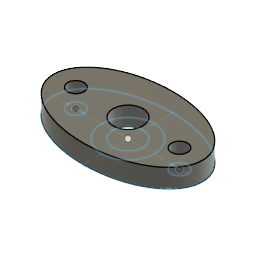
Assembled Box (Autodesk Fusion 360 archive; units mm, degrees)
design "Elllipse"
part number: 2026-06-03-15-20-48-513
Autodesk Fusion 360 part; units mm, degrees
sketch "Sketch1" plane through (0, 0, 0) normal (0, 1, 0) x (1, 0, 0)
sketch "Sketch2" plane through (0, 15, 0) normal (0, 1, 0) x (-1, 0, 0)
sketch "Sketch3" plane through (0, 15, 0) normal (0, 1, 0) x (-1, 0, 0)
  ellipse E0 centre (250.1558, -249.9936) end of major axis (250.1558, -285.9936) minor radius 60
  line L0 (250.1558, -213.9936) -> (250.1558, -285.9936) construction
  line L1 (190.1558, -249.9936) -> (310.1558, -249.9936) construction
  line L2 (214.6588, -249.4953) -> (208.1588, -249.4953)
  circle A0 centre (208.1588, -249.4953) radius 6.5
  line L3 (285.6558, -249.9936) -> (292.1558, -249.9936)
  circle A1 centre (292.1558, -249.9936) radius 6.5
  circle A2 centre (250.1558, -249.9936) radius 12
  circle A3 centre (250.1558, -249.9936) radius 21
  dimension "d14" = 72
  dimension "d15" = 120
  dimension "d16" = 42
  dimension "d17" = 13
  dimension "d18" = 42
  dimension "d19" = 13
  dimension "d24" = 24
  dimension "d25" = 42
  constraint coincident E0 L0.start
  constraint coincident E0 L0.end
  constraint coincident E0 L1.start
  constraint coincident E0 L1.end
  constraint vertical L0
  constraint perpendicular L0 L2
  constraint coincident L2.end A0.centre
  constraint perpendicular L0 L3
  constraint coincident L3.end A1.centre
  constraint coincident A1 L3.start
  constraint coincident A0 L2.start
  constraint concentric E0 A2
  constraint concentric E0 A3
  measures "d14" distance of E0
  measures "d16" distance of E0.centre L2.end
  measures "d17" diameter of A0
  measures "d18" distance of E0.centre L3.end
  measures "d19" diameter of A1
  measures "d24" diameter of A2
  measures "d25" diameter of A3
extrude "Extrude3" add sketch "Sketch3" along normal blind 15 contours E0 | A3
sketch "Sketch4" plane through (0, 0, 0) normal (0, 1, 0) x (1, 0, 0)
sketch "Sketch5" plane through (0, 0, 0) normal (0, 1, 0) x (1, 0, 0)

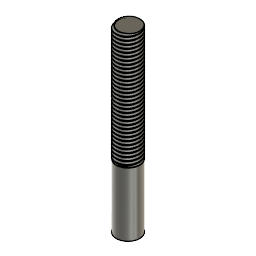
design "rod maker"
part number: 2026-06-04-10-37-24-051
Autodesk Fusion 360 part; units mm, degrees
sketch "Sketch1" plane through (0, 0, 0) normal (1, 0, 0) x (0, 1, 0)
sketch "Sketch2" plane through (0, 0, 0) normal (0, 0, 1) x (1, 0, 0)
sketch "Sketch3" plane through (0, 0, 0) normal (0, 0, 1) x (1, 0, 0)
  circle A0 centre (0, 0) radius 6
  dimension "d1" = 12
  constraint coincident A0.centre origin
  measures "d1" diameter of A0
extrude "Extrude1" add sketch "Sketch3" along normal blind 70
sketch "Sketch4" plane through (0, 0, 0) normal (1, 0, 0) x (0, 1, 0)
thread "Thread1" "ISO Metric profile 12.0 M12x1.75 M12x1.75 6g" major diameter 11.8335 minor diameter 9.8365 pitch 1.75 angle 60 modelled right hand crest width 0.2518 on face at (5.9702, -0.5974, 46.6667) from (0, 0, 12) to (0, 0, 70) crest through (5.9168, 0, -0.4375)
extrude "Extrude2" add 1 faces at (1.3581, 0.7601, 0) along direction (0, 0, -1) blind 20
named bodies: "rod maker"

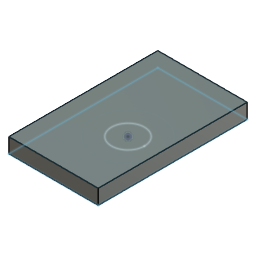
design "Bottom Plane"
part number: 2026-06-03-15-20-48-513
Autodesk Fusion 360 part; units mm, degrees
sketch "Sketch1" plane through (0, 0, 0) normal (0, 1, 0) x (1, 0, 0)
  line L0 (-45, 75) -> (-45, -75)
  line L1 (-45, -75) -> (45, -75)
  line L2 (45, -75) -> (45, 75)
  line L3 (45, 75) -> (-45, 75)
  circle A0 centre (0, 0) radius 16.5
  dimension "d9" = 33
  constraint perpendicular L0 L1
  constraint perpendicular L1 L2
  constraint coincident A0.centre origin
  measures "d9" diameter of A0
extrude "Extrude1" add sketch "Sketch1" along normal blind 15 contours L0 L1 L2 L3 | A0
move_face "MoveFace1" by (-220, 0, 0) 1 faces at (-15, 15, -25)
sketch "Sketch2" plane through (0, 15, 0) normal (0, 1, 0) x (-1, 0, 0)
  line L0 (-45, -75) -> (45, -75)
  line L1 (45, -75) -> (45, 75)
  line L2 (45, 75) -> (-45, 75)
  line L3 (-45, 75) -> (-45, -75)
sketch "Sketch3" plane through (0, 15, 0) normal (0, 1, 0) x (-1, 0, 0)
  line L0 (-45, -75) -> (45, -75)
  line L1 (45, -75) -> (45, 75)
  line L2 (45, 75) -> (-45, 75)
  line L3 (-45, 75) -> (-45, -75)
sketch "Sketch6" plane through (0, 30, 0) normal (0, 1, 0) x (-1, 0, 0)
sketch "Sketch10" plane through (0, 15, 0) normal (0, 1, 0) x (-1, 0, 0)
combine "Combine1" [no effect]
sketch "Sketch7" plane through (0, 15, 0) normal (0, 1, 0) x (-1, 0, 0)
sketch "Sketch8" plane through (0, 15, 0) normal (0, 1, 0) x (-1, 0, 0)
sketch "Sketch9" plane through (0, 15, 0) normal (0, 1, 0) x (-1, 0, 0)
extrude "Extrude3" [suppressed]
sketch "Sketch4" plane through (0, 0, 0) normal (0, 1, 0) x (1, 0, 0)
sketch "Sketch5" plane through (0, 0, 0) normal (0, 1, 0) x (1, 0, 0)
named bodies: "Body 1"

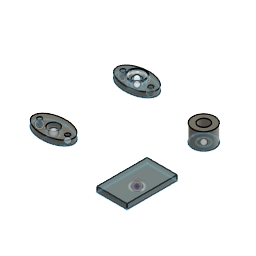
design "Stuffing Box"
part number: 2026-06-03-15-20-48-513
Autodesk Fusion 360 part; units mm, degrees
sketch "Sketch1" plane through (0, 0, 0) normal (0, 1, 0) x (1, 0, 0)
  line L0 (-45, 75) -> (-45, -75)
  line L1 (-45, -75) -> (45, -75)
  line L2 (45, -75) -> (45, 75)
  line L3 (45, 75) -> (-45, 75)
  circle A0 centre (0, 0) radius 16.5
  dimension "d9" = 33
  constraint perpendicular L0 L1
  constraint perpendicular L1 L2
  constraint coincident A0.centre origin
  measures "d9" diameter of A0
extrude "Extrude1" add sketch "Sketch1" along normal blind 15 contours L0 L1 L2 L3 | A0 makes body 1
move_face "MoveFace1" by (-220, 0, 0) 1 faces at (-15, 15, -25) on bodies 1
sketch "Sketch2" plane through (0, 15, 0) normal (0, 1, 0) x (-1, 0, 0)
  line L0 (-45, -75) -> (45, -75)
  line L1 (45, -75) -> (45, 75)
  line L2 (45, 75) -> (-45, 75)
  line L3 (-45, 75) -> (-45, -75)
  circle A0 centre (0, -200) radius 33
  circle A1 centre (0, -200) radius 16.5
  dimension "d10" = 66
  dimension "d11" = 33
  constraint concentric A0 A1
  measures "d10" diameter of A0
  measures "d11" diameter of A1
extrude "Extrude2" add sketch "Sketch2" along normal blind 50 separate body contours A0 makes body 2
sketch "Sketch3" plane through (0, 15, 0) normal (0, 1, 0) x (-1, 0, 0)
  line L0 (-45, -75) -> (45, -75)
  line L1 (45, -75) -> (45, 75)
  line L2 (45, 75) -> (-45, 75)
  line L3 (-45, 75) -> (-45, -75)
  ellipse E0 centre (250.1558, -249.9936) end of major axis (250.1558, -285.9936) minor radius 60
  line L4 (250.1558, -213.9936) -> (250.1558, -285.9936) construction
  line L5 (190.1558, -249.9936) -> (310.1558, -249.9936) construction
  line L6 (214.6588, -249.4953) -> (208.1588, -249.4953)
  circle A0 centre (208.1588, -249.4953) radius 6.5
  line L7 (285.6558, -249.9936) -> (292.1558, -249.9936)
  circle A1 centre (292.1558, -249.9936) radius 6.5
  ellipse E1 centre (250, 0) end of major axis (250, -36) minor radius 60
  line L8 (250, 36) -> (250, -36) construction
  line L9 (190, 0) -> (310, 0) construction
  circle A2 centre (250, 0) radius 16.5
  circle A3 centre (250.1558, -249.9936) radius 12
  circle A4 centre (250.1558, -249.9936) radius 21
  circle A5 centre (208, 0) radius 6.5
  line L10 (250, 0) -> (292, 0) construction
  circle A6 centre (292, 0) radius 6.5
  dimension "d14" = 72
  dimension "d15" = 120
  dimension "d16" = 42
  dimension "d17" = 13
  dimension "d18" = 42
  dimension "d19" = 13
  dimension "d20" = 72
  dimension "d21" = 120
  dimension "d22" = 42
  dimension "d23" = 33
  dimension "d24" = 24
  dimension "d25" = 42
  dimension "d41" = 13
  dimension "d48" = 42
  dimension "d49" = 13
  constraint coincident E0 L4.start
  constraint coincident E0 L4.end
  constraint coincident E0 L5.start
  constraint coincident E0 L5.end
  constraint vertical L4
  constraint perpendicular L4 L6
  constraint coincident L6.end A0.centre
  constraint perpendicular L4 L7
  constraint coincident L7.end A1.centre
  constraint coincident A1 L7.start
  constraint coincident A0 L6.start
  constraint coincident E1 L8.start
  constraint coincident E1 L8.end
  constraint coincident E1 L9.start
  constraint coincident E1 L9.end
  constraint vertical L8
  constraint concentric E1 A2
  constraint concentric E0 A3
  constraint concentric E0 A4
  constraint coincident E1.centre A2.centre
  constraint perpendicular L8 L10
  constraint coincident L10.end A6.centre
  measures "d14" distance of E0
  measures "d16" distance of E0.centre L6.end
  measures "d17" diameter of A0
  measures "d18" distance of E0.centre L7.end
  measures "d19" diameter of A1
  measures "d20" distance of E1
  measures "d22" distance of E1.centre A5.centre
  measures "d23" diameter of A2
  measures "d24" diameter of A3
  measures "d25" diameter of A4
  measures "d41" diameter of A5
  measures "d48" distance of E1.centre L10.end
  measures "d49" diameter of A6
extrude "Extrude4" add sketch "Sketch3" along normal blind 15 separate body contours E0 makes body 3
extrude "Extrude5" add sketch "Sketch3" along normal blind 9 separate body contours A4 makes body 4
extrude "Extrude6" add 1 faces at (-268.033, 24, -251.633) along direction (0, 1, 0) blind 6 on bodies 4 bodies 3 4
sketch "Sketch6" plane through (0, 30, 0) normal (0, 1, 0) x (-1, 0, 0)
  circle A0 centre (250.1558, -249.9936) radius 12
  circle A1 centre (208.1588, -249.4953) radius 6.5
  circle A2 centre (292.1558, -249.9936) radius 6.5
  ellipse E0 centre (250.1558, -249.9936) end of major axis (310.1558, -249.9936) minor radius 36
  circle A3 centre (250.1558, -249.9936) radius 25
  circle A4 centre (250.1558, -249.9936) radius 23
  dimension "d35" = 50
  dimension "d36" = 46
  constraint concentric A0 A3
  constraint concentric A3 A4
  measures "d35" diameter of A3
  measures "d36" diameter of A4
extrude "Extrude7" add sketch "Sketch6" along normal blind 9 contours A3 bodies 3
fillet "Fillet1" radius 13.5 1 edges at (-228.7123, 30, -258.3107) on bodies 3
sketch "Sketch10" plane through (0, 15, 0) normal (0, 1, 0) x (-1, 0, 0)
extrude "Extrude9" add sketch "Sketch3" along normal blind 15 separate body contours E0 makes body 5
extrude "Extrude10" add sketch "Sketch3" along normal blind 15 separate body contours E1 makes body 6
combine "Combine1" operation add target body 3 tool bodies 5
sketch "Sketch7" plane through (0, 15, 0) normal (0, 1, 0) x (-1, 0, 0)
  line L0 (250, 0) -> (292, 0) construction
  circle A0 centre (292, 0) radius 6.5
  dimension "d42" = 42
  dimension "d43" = 13
  constraint horizontal L0
  constraint coincident L0.end A0.centre
  measures "d42" distance of L0.start L0.end
  measures "d43" diameter of A0
sketch "Sketch8" plane through (0, 15, 0) normal (0, 1, 0) x (-1, 0, 0)
extrude "Extrude8" add sketch "Sketch3" along normal blind 15 separate body contours E1 | A6 makes body 7
sketch "Sketch9" plane through (0, 15, 0) normal (0, 1, 0) x (-1, 0, 0)
extrude "Extrude3" [suppressed]
sketch "Sketch4" plane through (0, 0, 0) normal (0, 1, 0) x (1, 0, 0)
sketch "Sketch5" plane through (0, 0, 0) normal (0, 1, 0) x (1, 0, 0)
named bodies: "Body 1", "Body 2", "Body 3", "Body 4"

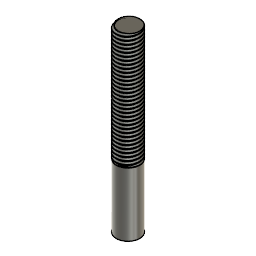
design "rod maker"
part number: 2026-06-04-10-37-24-051
Autodesk Fusion 360 part; units mm, degrees
sketch "Sketch1" plane through (0, 0, 0) normal (1, 0, 0) x (0, 1, 0)
sketch "Sketch2" plane through (0, 0, 0) normal (0, 0, 1) x (1, 0, 0)
sketch "Sketch3" plane through (0, 0, 0) normal (0, 0, 1) x (1, 0, 0)
  circle A0 centre (0, 0) radius 6
  dimension "d1" = 12
  constraint coincident A0.centre origin
  measures "d1" diameter of A0
extrude "Extrude1" add sketch "Sketch3" along normal blind 70
sketch "Sketch4" plane through (0, 0, 0) normal (1, 0, 0) x (0, 1, 0)
thread "Thread1" "ISO Metric profile 12.0 M12x1.75 M12x1.75 6g" major diameter 11.8335 minor diameter 9.8365 pitch 1.75 angle 60 modelled right hand crest width 0.2518 on face at (5.9702, -0.5974, 46.6667) from (0, 0, 12) to (0, 0, 70) crest through (5.9168, 0, -0.4375)
extrude "Extrude2" add 1 faces at (1.3581, 0.7601, 0) along direction (0, 0, -1) blind 20

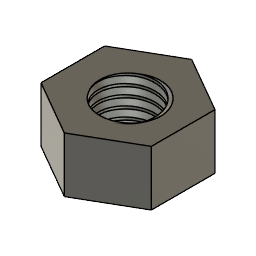
design "nut"
part number: 2026-06-04-11-31-36-315
Autodesk Fusion 360 part; units mm, degrees
sketch "Sketch1" plane through (0, 0, 0) normal (0, 0, 1) x (1, 0, 0)
  circle A0 centre (0, 0) radius 6
  line L0 (10, 5.7735) -> (0, 11.547)
  line L1 (0, 11.547) -> (-10, 5.7735)
  line L2 (-10, 5.7735) -> (-10, -5.7735)
  line L3 (-10, -5.7735) -> (0, -11.547)
  line L4 (0, -11.547) -> (10, -5.7735)
  line L5 (10, -5.7735) -> (10, 5.7735)
  dimension "d3" = 12
  constraint coincident A0.centre origin
  measures "d3" diameter of A0
extrude "Extrude1" add sketch "Sketch1" along normal blind 10
thread "Thread1" "ISO Metric profile 12.0 M12x1.75 M12x1.75 6H" major diameter 12.2265 minor diameter 10.2735 pitch 1.75 angle 60 modelled right hand crest width 0.4769 on face at (5.9925, -0.2991, 6.6667) crest through (5.1368, 0, 0.4375)

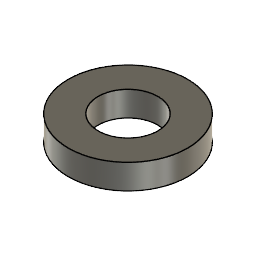
design "Screw"
part number: 2026-06-04-11-09-47-763
Autodesk Fusion 360 part; units mm, degrees
sketch "Sketch1" plane through (0, 0, 0) normal (1, 0, 0) x (0, 1, 0)
  line L0 (0, 0) -> (0, 5)
  line L1 (6, 0) -> (12, 0)
  line L2 (12, 0) -> (12, 5)
  line L3 (12, 5) -> (6, 5)
  line L4 (6, 5) -> (6, 0)
  dimension "d7" = 5
  dimension "d8" = 6
  constraint coincident L0.start origin
  constraint vertical L0
  constraint perpendicular L1 L2
  constraint perpendicular L2 L3
  measures "d7" distance of L0.start L0.end
  measures "d8" distance of L1.start L1.end
revolve "Revolve1" add sketch "Sketch1" angle 360 about axis through (0, 0, 0) along (0, 0, 1)
named bodies: "rod bottom cap"

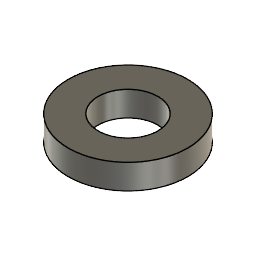
design "Screw"
part number: 2026-06-04-11-09-47-763
Autodesk Fusion 360 part; units mm, degrees
sketch "Sketch1" plane through (0, 0, 0) normal (1, 0, 0) x (0, 1, 0)
  line L0 (0, 0) -> (0, 5)
  line L1 (6, 0) -> (12, 0)
  line L2 (12, 0) -> (12, 5)
  line L3 (12, 5) -> (6, 5)
  line L4 (6, 5) -> (6, 0)
  dimension "d7" = 5
  dimension "d8" = 6
  constraint coincident L0.start origin
  constraint vertical L0
  constraint perpendicular L1 L2
  constraint perpendicular L2 L3
  measures "d7" distance of L0.start L0.end
  measures "d8" distance of L1.start L1.end
revolve "Revolve1" add sketch "Sketch1" angle 360 about axis through (0, 0, 0) along (0, 0, 1)

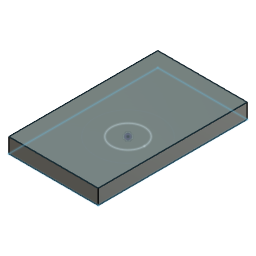
design "Stuffing Box"
part number: 2026-06-03-15-20-48-513
Autodesk Fusion 360 part; units mm, degrees
sketch "Sketch1" plane through (0, 0, 0) normal (0, 1, 0) x (1, 0, 0)
  line L0 (-45, 75) -> (-45, -75)
  line L1 (-45, -75) -> (45, -75)
  line L2 (45, -75) -> (45, 75)
  line L3 (45, 75) -> (-45, 75)
  circle A0 centre (0, 0) radius 16.5
  dimension "d9" = 33
  constraint perpendicular L0 L1
  constraint perpendicular L1 L2
  constraint coincident A0.centre origin
  measures "d9" diameter of A0
extrude "Extrude1" add sketch "Sketch1" along normal blind 15 contours L0 L1 L2 L3 | A0
move_face "MoveFace1" by (-220, 0, 0) 1 faces at (-15, 15, -25)
sketch "Sketch2" plane through (0, 15, 0) normal (0, 1, 0) x (-1, 0, 0)
  line L0 (-45, -75) -> (45, -75)
  line L1 (45, -75) -> (45, 75)
  line L2 (45, 75) -> (-45, 75)
  line L3 (-45, 75) -> (-45, -75)
sketch "Sketch3" plane through (0, 15, 0) normal (0, 1, 0) x (-1, 0, 0)
  line L0 (-45, -75) -> (45, -75)
  line L1 (45, -75) -> (45, 75)
  line L2 (45, 75) -> (-45, 75)
  line L3 (-45, 75) -> (-45, -75)
sketch "Sketch6" plane through (0, 30, 0) normal (0, 1, 0) x (-1, 0, 0)
sketch "Sketch10" plane through (0, 15, 0) normal (0, 1, 0) x (-1, 0, 0)
combine "Combine1" [no effect]
sketch "Sketch7" plane through (0, 15, 0) normal (0, 1, 0) x (-1, 0, 0)
sketch "Sketch8" plane through (0, 15, 0) normal (0, 1, 0) x (-1, 0, 0)
sketch "Sketch9" plane through (0, 15, 0) normal (0, 1, 0) x (-1, 0, 0)
extrude "Extrude3" [suppressed]
sketch "Sketch4" plane through (0, 0, 0) normal (0, 1, 0) x (1, 0, 0)
sketch "Sketch5" plane through (0, 0, 0) normal (0, 1, 0) x (1, 0, 0)
named bodies: "Body 1"

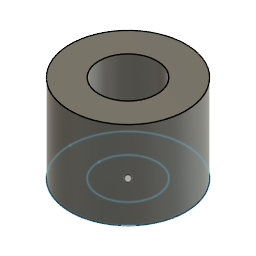
design "Cylinder"
part number: 2026-06-03-15-20-48-513
Autodesk Fusion 360 part; units mm, degrees
sketch "Sketch1" plane through (0, 0, 0) normal (0, 1, 0) x (1, 0, 0)
sketch "Sketch2" plane through (0, 15, 0) normal (0, 1, 0) x (-1, 0, 0)
  circle A0 centre (0, -200) radius 33
  circle A1 centre (0, -200) radius 16.5
  dimension "d10" = 66
  dimension "d11" = 33
  constraint concentric A0 A1
  measures "d10" diameter of A0
  measures "d11" diameter of A1
extrude "Extrude2" add sketch "Sketch2" along normal blind 50
sketch "Sketch3" plane through (0, 15, 0) normal (0, 1, 0) x (-1, 0, 0)
sketch "Sketch4" plane through (0, 0, 0) normal (0, 1, 0) x (1, 0, 0)
sketch "Sketch5" plane through (0, 0, 0) normal (0, 1, 0) x (1, 0, 0)
